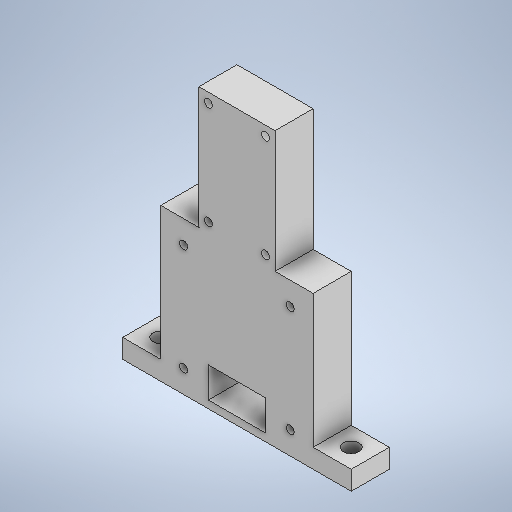
# Autodesk Inventor part: camera_new
Saved by Autodesk Inventor 2026.1 (Build 301233000, 233)
## iProperties
Created: 2026-05-25
Part Number: camera_new
Material: Generic
Document SubType Name: Modeling
Designer: chris
Density: 1 g/cm^3
Appearance: Default
Author: chris
Autodesk Inventor part; units mm, degrees
ref_plane "YZ Plane" through (0, 0, 0) normal (1, 0, 0) x (0, 1, 0)
ref_plane "XZ Plane" through (0, 0, 0) normal (0, 1, 0) x (-1, 0, 0)
ref_plane "XY Plane" through (0, 0, 0) normal (0, 0, 1) x (1, 0, 0)
sketch "Sketch1" plane through (0, 0, 0) normal (0, 0, 1) x (1, 0, 0)
  line L0 (-20, -20) -> (20, -20)
  line L1 (20, -20) -> (20, 20)
  line L2 (20, 20) -> (-20, 20)
  line L3 (-20, 20) -> (-20, -20)
  line L4 (-20, -20) -> (20, 20) construction
  line L5 (20, -20) -> (-20, 20) construction
  point P0 (0, 0)
  dimension "d0" = 40
  dimension "d1" = 40
  constraints: 12 end point, 2 midpoint, 2 parallel, 1 horizontal, 1 perpendicular
  measures "d0" distance of L2.end L1.end
  measures "d1" distance of L1.end L0.end
extrude "Extrusion1" add sketch "Sketch1" along normal blind 10
sketch "Sketch2" plane through (0, 0, 10) normal (0, 0, 1) x (1, 0, 0)
  circle A0 centre (-14, 14) radius 1.05
  circle A1 centre (-14, -14) radius 1.05
  circle A2 centre (14, -14) radius 1.05
  circle A3 centre (14, 14) radius 1.05
  point P0 (0, 0)
  dimension "d4" = 2.1
  dimension "d5" = 2.1
  dimension "d6" = 2.1
  dimension "d7" = 2.1
  dimension "d8" = 14
  dimension "d9" = 14
  dimension "d10" = 14
  dimension "d11" = 14
  constraints: 4 centre point, 2 horizontal alignment, 2 vertical alignment
  measures "d4" diameter of A0
  measures "d5" diameter of A1
  measures "d6" diameter of A2
  measures "d7" diameter of A3
  measures "d8" horizontal distance of A1.centre point (0, 0)
  measures "d9" horizontal distance of A2.centre point (0, 0)
  measures "d10" horizontal distance of A3.centre point (0, 0)
  measures "d11" horizontal distance of A2.centre point (0, 0)
extrude "Extrusion2" cut sketch "Sketch2" against normal blind 10
sketch "Sketch3" plane through (0, 0, 10) normal (0, 0, 1) x (1, 0, 0)
  line L0 (-7.5, -18) -> (7.5, -18)
  line L1 (7.5, -18) -> (7.5, -10)
  line L2 (7.5, -10) -> (-7.5, -10)
  line L3 (-7.5, -10) -> (-7.5, -18)
  line L4 (-7.5, -18) -> (7.5, -10) construction
  line L5 (7.5, -18) -> (-7.5, -10) construction
  point P0 (0, 0)
  point P1 (0, -14)
  dimension "d14" = 15
  dimension "d15" = 8
  dimension "d16" = 14
  constraints: 12 end point, 2 midpoint, 2 parallel, 1 horizontal, 1 perpendicular
  measures "d14" distance of L2.end L1.end
  measures "d15" distance of L1.end L0.end
  measures "d16" distance of point (0, -14) point (0, 0)
extrude "Extrusion3" cut sketch "Sketch3" against normal blind 10
sketch "Sketch4" plane through (-20, -20, 0) normal (0, -1, 0) x (1, 0, 0)
  line L0 (0, 0) -> (-10, 0)
  line L1 (-10, 0) -> (-10, 10)
  line L2 (-10, 10) -> (0, 10)
  line L3 (0, 10) -> (0, 0)
  line L4 (50, 0) -> (40, 0)
  line L5 (40, 0) -> (40, 10)
  line L6 (40, 10) -> (50, 10)
  line L7 (50, 10) -> (50, 0)
  line L8 (0, 0) -> (0, 10) projected
  line L9 (40, 0) -> (40, 10) projected
  line L10 (0, 0) -> (40, 0) projected
  line L11 (0, 10) -> (40, 10) projected
  point P0 (20, 0)
  dimension "d19" = 10
  dimension "d20" = 10
  constraints: 16 end point, 5 collinear, 4 parallel, 2 horizontal, 2 perpendicular, 1 point on line
  measures "d19" distance of L5.end L6.end
  measures "d20" distance of L1.end L2.end
extrude "Extrusion4" add sketch "Sketch4" against normal blind 5 contours L0 L1 L2 L3 | L5 L6 L7 L4
sketch "Sketch5" plane through (-20, -15, 0) normal (0, 1, 0) x (1, 0, 0)
  circle A0 centre (-5, -5) radius 2.05
  circle A1 centre (45, -5) radius 2.05
  line L0 (-10, 0) -> (-10, -10) projected
  line L1 (-10, -10) -> (0, -10) projected
  line L2 (50, 0) -> (40, 0) projected
  line L3 (50, -10) -> (50, 0) projected
  point P0 (20, 0)
  dimension "d23" = 4.1
  dimension "d24" = 4.1
  dimension "d25" = 5
  dimension "d26" = 5
  dimension "d27" = 5
  dimension "d28" = 5
  constraints: 2 centre point
  measures "d23" diameter of A0
  measures "d24" diameter of A1
  measures "d25" distance from line of L0 A0.centre
  measures "d26" distance from line of L1 A0.centre
  measures "d27" distance from line of L2 A1.centre
  measures "d28" distance from line of L3 A1.centre
extrude "Extrusion5" cut sketch "Sketch5" against normal blind 5
sketch "Sketch6" plane through (-20, 20, 0) normal (0, 1, 0) x (1, 0, 0)
  line L0 (30, -10) -> (10, -10)
  line L1 (10, -10) -> (10, 0)
  line L2 (10, 0) -> (30, 0)
  line L3 (30, 0) -> (30, -10)
  line L4 (40, -10) -> (0, -10) projected
  line L5 (40, 0) -> (40, -10) projected
  line L6 (40, 0) -> (0, 0) projected
  line L7 (0, 0) -> (0, -10) projected
  point P0 (20, 0)
  dimension "d33" = 20
  dimension "d34" = 10
  constraints: 8 end point, 2 collinear, 2 parallel, 1 horizontal, 1 perpendicular
  measures "d33" distance between parallel lines of L3 L1
  measures "d34" distance between parallel lines of L5 L3
extrude "Extrusion6" add sketch "Sketch6" along normal blind 32 contours L0 L1 L2 L3
sketch "Sketch7" plane through (0, 0, 0) normal (0, 0, -1) x (-1, 0, 0)
  circle A0 centre (-7.5, 49.5) radius 1.05
  circle A1 centre (-7.5, 22.5) radius 1.05
  circle A2 centre (7.5, 49.5) radius 1.05
  circle A3 centre (7.5, 22.5) radius 1.05
  line L0 (-10, 52) -> (10, 52) projected
  line L1 (-10, 20) -> (-10, 52) projected
  point P0 (0, 0)
  dimension "d35" = 2.1
  dimension "d36" = 2.1
  dimension "d37" = 2.1
  dimension "d38" = 2.1
  dimension "d39" = 15
  dimension "d40" = 27
  dimension "d41" = 2.5
  dimension "d42" = 2.5
  constraints: 4 centre point, 2 horizontal alignment, 2 vertical alignment
  measures "d35" diameter of A0
  measures "d36" diameter of A1
  measures "d37" diameter of A2
  measures "d38" diameter of A3
  measures "d39" distance of A2.centre A0.centre
  measures "d40" distance of A1.centre A0.centre
  measures "d41" distance from line of L0 A0.centre
  measures "d42" distance from line of L1 A0.centre
extrude "Extrusion7" cut sketch "Sketch7" against normal blind 32
body "Solid1"
